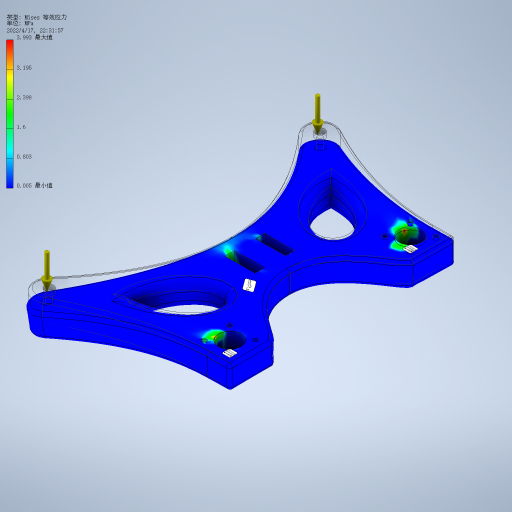
# Autodesk Inventor part: Z托架
Saved by Autodesk Inventor 2023 (Build 270158000, 158)
## iProperties
Created: 2022-04-17
Part Number: Z托架
Material: ABS 塑料
Document SubType Name: Modeling
Designer: Zhong
Density: 1.06 g/cm^3
Appearance: 平滑 - 白色
Mass: 162.237 g
Surface Area: 365.398 cm^2
Volume: 153.054 cm^3
Author: Zhong
Autodesk Inventor part; units mm, degrees
ref_plane "YZ Plane" through (0, 0, 0) normal (1, 0, 0) x (0, 1, 0)
ref_plane "XZ Plane" through (0, 0, 0) normal (0, 1, 0) x (-1, 0, 0)
ref_plane "XY Plane" through (0, 0, 0) normal (0, 0, 1) x (1, 0, 0)
sketch "草图1" plane through (0, 0, 0) normal (0, 1, 0) x (-1, 0, 0)
  line L0 (-13, 75) -> (0, 75)
  line L1 (-15, 47) -> (-15, 73)
  circle A0 centre (0, 60) radius 7.55
  line L2 (50, 13) -> (30, 13)
  line L3 (30, 13) -> (30, 7)
  line L4 (30, 7) -> (50, 7)
  line L5 (50, 7) -> (50, 13)
  line L6 (50, 13) -> (30, 7) construction
  line L7 (30, 13) -> (50, 7) construction
  line L8 (-15, 0) -> (135, 0) construction
  arc A1 (97.5655, 83.4607) -> (85.3449, 98.8504) centre (90, 90) ccw
  line L9 (0, 75) -> (40, 75) construction
  line L10 (40, 75) -> (85.3449, 98.8504) construction
  spline S0 degree 2 poles (0, 75) (40, 75) (85.3449, 98.8504) knots 1 1 1 2 2 2
  line L11 (60, 0) -> (60, 40) construction
  line L12 (60, 40) -> (97.5655, 83.4607) construction
  spline S1 degree 2 poles (60, 0) (60, 40) (97.5655, 83.4607) knots 1 1 1 2 2 2
  arc A2 (-13, 75) -> (-15, 73) centre (-13, 73) ccw
  circle A3 centre (8.5, 68.5) radius 1.55
  circle A4 centre (-8.5, 68.5) radius 1.55
  circle A5 centre (-8.5, 51.5) radius 1.55
  circle A6 centre (8.5, 51.5) radius 1.55
  line L13 (-13, -75) -> (0, -75)
  line L14 (-15, -47) -> (-15, -73)
  circle A7 centre (0, -60) radius 7.55
  line L15 (50, -13) -> (30, -13)
  line L16 (30, -13) -> (30, -7)
  line L17 (30, -7) -> (50, -7)
  line L18 (50, -7) -> (50, -13)
  line L19 (50, -13) -> (30, -7) construction
  line L20 (30, -13) -> (50, -7) construction
  arc A8 (85.3449, -98.8504) -> (97.5655, -83.4607) centre (90, -90) ccw
  line L21 (0, -75) -> (40, -75) construction
  line L22 (40, -75) -> (85.3449, -98.8504) construction
  spline S2 degree 2 poles (0, -75) (40, -75) (85.3449, -98.8504) knots 1 1 1 2 2 2
  line L23 (60, 0) -> (60, -40) construction
  line L24 (60, -40) -> (97.5655, -83.4607) construction
  spline S3 degree 2 poles (60, 0) (60, -40) (97.5655, -83.4607) knots 1 1 1 2 2 2
  arc A9 (-15, -73) -> (-13, -75) centre (-13, -73) ccw
  circle A10 centre (8.5, -68.5) radius 1.55
  circle A11 centre (-8.5, -68.5) radius 1.55
  circle A12 centre (-8.5, -51.5) radius 1.55
  circle A13 centre (8.5, -51.5) radius 1.55
  line L25 (90, 90) -> (0, -60) construction
  line L26 (0, 60) -> (0, -60) construction
  line L27 (40, 0) -> (0, 60) construction
  line L28 (-15, 47) -> (-15, 40) construction
  line L29 (-15, 40) -> (20, 30) construction
  line L30 (20, 30) -> (20, 0) construction
  spline S4 degree 3 poles (-15, 47) (-15, 40) (20, 30) (20, 0) knots 1 1 1 1 2 2 2 2
  line L31 (60, 66.95) -> (0, 60) construction
  line L32 (0, 60) -> (20, 0) construction
  line L33 (20, 0) -> (60, 40) construction
  line L34 (60, 40) -> (60, 66.95) construction
  spline S5 degree 4 poles (60, 66.95) (0, 60) (20, 0) (60, 40) (60, 66.95) knots 1 1 1 1 1 2 2 2 2 2
  line L35 (-15, -47) -> (-15, -40) construction
  line L36 (-15, -40) -> (20, -30) construction
  line L37 (20, -30) -> (20, 0) construction
  spline S6 degree 3 poles (-15, -47) (-15, -40) (20, -30) (20, 0) knots 1 1 1 1 2 2 2 2
  line L38 (60, -66.95) -> (0, -60) construction
  line L39 (0, -60) -> (20, 0) construction
  line L40 (20, 0) -> (60, -40) construction
  line L41 (60, -40) -> (60, -66.95) construction
  spline S7 degree 4 poles (60, -66.95) (0, -60) (20, 0) (60, -40) (60, -66.95) knots 1 1 1 1 1 2 2 2 2 2
  point P0 (0, 0)
  point P1 (-15, 75)
  point P2 (40, 10)
  point P3 (-15, -75)
  point P4 (40, -10)
  dimension "d2" = 15.1
  dimension "d6" = 20
  dimension "d7" = 6
  dimension "d8" = 40
  dimension "d9" = 20
  dimension "d10" = 120
  dimension "d11" = 150
  dimension "d12" = 15
  dimension "d13" = 180
  dimension "d15" = 20
  dimension "d16" = 20
  dimension "d17" = 2
  dimension "d18" = 3.1
  dimension "d19" = 8.5
  dimension "d20" = 8.5
  dimension "d23" = 360
  dimension "d26" = 28
  dimension "d31" = 20
  constraints: 40 end point, 26 symmetric about line, 14 centre point, 11 point on line, 8 point on circle, 5 midpoint, 4 coincident, 4 tangent, 3 horizontal, 2 parallel, 2 perpendicular, 2 vertical, 38 other
  measures "d2" diameter of A0
  measures "d6" distance of L2.start L2.end
  measures "d7" distance of L4.end L2.start
  measures "d8" horizontal distance of point (0, 0) point (40, 10)
  measures "d9" diameter of point (40, 10) L8
  measures "d10" diameter of L26.start L8
  measures "d11" diameter of point (-15, 75) L8
  measures "d12" distance of point (-15, 75) L0.end
  measures "d13" diameter of L25.start L8
  measures "d15" diameter of A1
  measures "d16" horizontal distance of point (40, 10) L11.start
  measures "d17" radius of A2
  measures "d18" diameter of A3
  measures "d19" horizontal distance of L26.start A3.centre
  measures "d20" horizontal distance of L26.start A3.centre
  measures "d26" distance of L1.start point (-15, 75)
  measures "d31" horizontal distance of L30.end point (40, 10)
extrude "拉伸1" add sketch "草图1" along normal blind 15
fillet "圆角1" radius 5 4 edges at (-30, 15, -33.3687) (-30, 0, -33.3687) (-30, 15, 33.3687) (-30, 0, 33.3687)
fillet "圆角2" radius 2 28 edges at (-69.3914, 15, -40.8652) (-69.3914, 15, 40.8652) (-97.8313, 15, 96.2186) (-41.3362, 15, 80.9626) (6.5, 15, 75) (14.4142, 15, 74.4142) (15, 15, 60) (-2.5, 15, 32.125) (-2.5, 15, -32.125) (15, 15, -60) (14.4142, 15, -74.4142) (6.5, 15, -75) (-41.3362, 15, -80.9626) (-97.8313, 15, -96.2186) (-69.3914, 0, 40.8652) (-97.8313, 0, 96.2186) (-41.3362, 0, 80.9626) (6.5, 0, 75) (14.4142, 0, 74.4142) (15, 0, 60) (-2.5, 0, 32.125) (-2.5, 0, -32.125) (15, 0, -60) (14.4142, 0, -74.4142) (6.5, 0, -75) (-41.3362, 0, -80.9626) (-97.8313, 0, -96.2186) (-69.3914, 0, -40.8652)
hole "孔1" at (-8.5, 0, 51.5) at (8.5, 0, 51.5) at (8.5, 0, -51.5) at (-8.5, 0, -51.5) at (8.5, 0, -68.5) at (-8.5, 0, -68.5) at (8.5, 0, 68.5) at (-8.5, 0, 68.5) direction (0, 1, 0) diameter 6 depth 5 tip angle 118
sketch "草图2" plane through (0, 15, 0) normal (0, 1, 0) x (1, 0, 0)
  arc A0 (-85.3449, 98.8504) -> (-97.5655, 83.4607) centre (-90, 90) ccw projected
  point P0 (0, 0)
  point P1 (-90, -90)
  dimension "d43" = 180
  constraints: 1 coincident
  measures "d43" distance of point (-90, -90) point (-90, 90)
hole "孔2" at (-90, 15, -90) at (-90, 15, 90) direction (0, -1, 0) diameter 3.1 end through all counterbore diameter 6 counterbore depth 3
